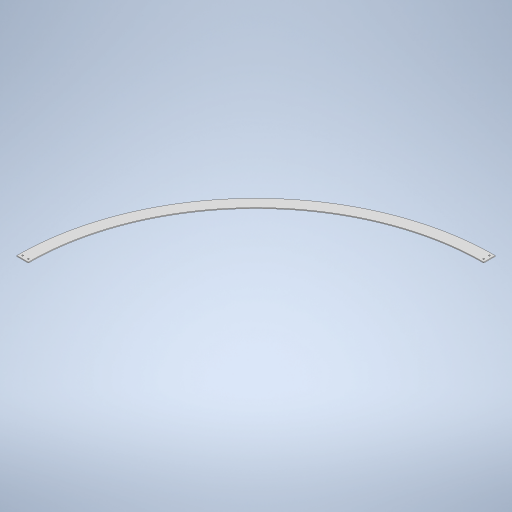
# Autodesk Inventor part: Arco menor
Saved by Autodesk Inventor 2024 (Build 280153000, 153)
## iProperties
Created: 2024-05-02
Part Number: Arco menor
Material: Genérico
Document SubType Name: Modeling
Designer: mathe
Density: 1 g/cm^3
Appearance: Padrão
Author: mathe
Autodesk Inventor part; units mm, degrees
ref_plane "YZ Plane" through (0, 0, 0) normal (1, 0, 0) x (0, 1, 0)
ref_plane "XZ Plane" through (0, 0, 0) normal (0, 1, 0) x (-1, 0, 0)
ref_plane "XY Plane" through (0, 0, 0) normal (0, 0, 1) x (1, 0, 0)
sketch "Esboço1" plane through (0, 0, 0) normal (0, 1, 0) x (-1, 0, 0)
  arc A0 (0, -800) -> (800, 0) centre (0, 0) ccw
  arc A1 (0, -840) -> (840, 0) centre (0, 0) ccw
  line L0 (800, 0) -> (840, 0)
  line L1 (0, -800) -> (0, -840)
  circle A2 centre (10, -810) radius 2.5
  circle A3 centre (10, -830) radius 2.5
  circle A4 centre (830, -10) radius 2.5
  circle A5 centre (810, -10) radius 2.5
  circle A6 centre (830, -10) radius 2.5
  circle A7 centre (810, -10) radius 2.5
  dimension "d0" = 800
  dimension "d1" = 840
  dimension "d2" = 5
  dimension "d3" = 5
  dimension "d4" = 20
  dimension "d6" = 10
  dimension "d7" = 5
  dimension "d8" = 5
  dimension "d9" = 10
  dimension "d10" = 10
  dimension "d11" = 20
  dimension "d13" = 10
  dimension "d14" = 10
  dimension "d15" = 10
  constraints: 8 centre point, 4 coincident, 4 end point, 4 point on circle, 2 concentric, 1 horizontal, 1 perpendicular
  measures "d0" radius of A0
  measures "d1" radius of A1
  measures "d2" diameter of A2
  measures "d3" diameter of A3
  measures "d4" distance of A3.centre A2.centre
  measures "d6" distance from line of L1 A2.centre
  measures "d7" diameter of A4
  measures "d8" diameter of A5
  measures "d9" distance from line of L0 A5.centre
  measures "d10" horizontal distance of L0.end A4.centre
  measures "d11" distance of A5.centre A4.centre
  measures "d13" distance from line of L0 A4.centre
  measures "d14" distance from line of L1 A3.centre
  measures "d15" horizontal distance of L1.end A3.centre
extrude "Extrusão1" add sketch "Esboço1" along normal blind 3 contours A0 L0 A1 L1 | A2 | A3 | A4 | A5
sketch "Esboço4" plane through (0, 3, 0) normal (0, 1, 0) x (1, 0, 0)
  circle A0 centre (-830, 10) radius 2.5
  circle A1 centre (-810, 10) radius 2.5
  line L0 (-840, 0) -> (-800, 0) projected
  circle A2 centre (-10, 810) radius 2.5
  circle A3 centre (-10, 830) radius 2.5
  line L1 (0, 800) -> (0, 840) projected
  point P0 (0, 0)
  dimension "d18" = 5
  dimension "d19" = 5
  dimension "d20" = 20
  dimension "d21" = 10
  dimension "d22" = 10
  dimension "d23" = 10
  dimension "d24" = 5
  dimension "d25" = 5
  dimension "d26" = 10
  dimension "d27" = 10
  dimension "d28" = 20
  dimension "d29" = 10
  constraints: 4 centre point
  measures "d18" diameter of A0
  measures "d19" diameter of A1
  measures "d20" distance of A0.centre A1.centre
  measures "d21" distance from line of L0 A0.centre
  measures "d22" distance from line of L0 A1.centre
  measures "d23" horizontal distance of L0.start A0.centre
  measures "d24" diameter of A2
  measures "d25" diameter of A3
  measures "d26" distance from line of L1 A3.centre
  measures "d27" horizontal distance of L1.start A2.centre
  measures "d28" distance of A3.centre A2.centre
  measures "d29" horizontal distance of L1.start A2.centre
hole "Furo1" at (-830, 3, -10) at (-810, 3, -10) at (-10, 3, -810) at (-10, 3, -830) direction (0, -1, 0) diameter 5 end through all
